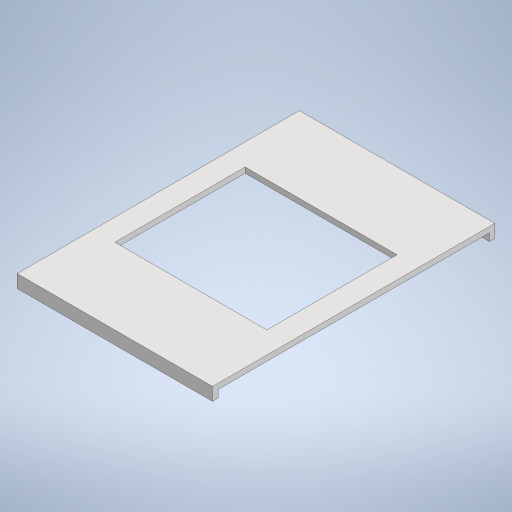
# Autodesk Inventor part: machine_platform
Saved by Autodesk Inventor 2024 (Build 280153000, 153)
## iProperties
Created: 2023-08-26
Part Number: machine_platform
Material: Generic
Document SubType Name: Modeling
Designer: l1534
Density: 1 g/cm^3
Appearance: Default
Author: l1534
Autodesk Inventor part; units mm, degrees
ref_plane "YZ Plane" through (0, 0, 0) normal (1, 0, 0) x (0, 1, 0)
ref_plane "XZ Plane" through (0, 0, 0) normal (0, 1, 0) x (-1, 0, 0)
ref_plane "XY Plane" through (0, 0, 0) normal (0, 0, 1) x (1, 0, 0)
sketch "Sketch1" plane through (0, 0, 0) normal (0, 1, 0) x (-1, 0, 0)
  line L0 (50.1781, 160.1313) -> (-129.8219, 160.1313)
  line L1 (-129.8219, 160.1313) -> (-129.8219, -99.8687)
  line L2 (-129.8219, -99.8687) -> (50.1781, -99.8687)
  line L3 (50.1781, -99.8687) -> (50.1781, 160.1313)
  point P0 (0, 0)
  dimension "d0" = 260
  dimension "d1" = 180
  constraints: 8 end point, 2 parallel, 1 horizontal, 1 perpendicular
  measures "d0" distance of L2.end L0.start
  measures "d1" distance of L1.end L2.end
extrude "Extrusion1" add sketch "Sketch1" along normal blind 5
sketch "Sketch2" plane through (0, 0, 0) normal (0, -1, 0) x (1, 0, 0)
  line L0 (129.8219, 160.1313) -> (129.8219, -99.8687) projected
  line L1 (-50.1781, -99.8687) -> (-50.1781, 160.1313) projected
  line L2 (129.8219, 160.1313) -> (-50.1781, 160.1313)
  line L3 (-50.1781, 160.1313) -> (-50.1781, 155.1313)
  line L4 (-50.1781, 155.1313) -> (129.8219, 155.1313)
  line L5 (129.8219, 155.1313) -> (129.8219, 160.1313)
  line L6 (129.8219, -99.8687) -> (-50.1781, -99.8687)
  line L7 (-50.1781, -99.8687) -> (-50.1781, -94.8687)
  line L8 (-50.1781, -94.8687) -> (129.8219, -94.8687)
  line L9 (129.8219, -94.8687) -> (129.8219, -99.8687)
  point P0 (0, 0)
  point P1 (129.8219, 155.1313)
  dimension "d4" = 5
  dimension "d5" = 5
  constraints: 16 end point, 4 parallel, 2 horizontal, 2 perpendicular, 2 point on line
  measures "d4" distance between parallel lines of L2 L4
  measures "d5" distance between parallel lines of L6 L8
extrude "Extrusion2" add sketch "Sketch2" along normal blind 7 contours L0 L4 L1 L2 | L0 L6 L1 L8
sketch "Sketch3" plane through (0, 5, 0) normal (0, 1, 0) x (1, 0, 0)
  line L0 (109.8219, 29.8687) -> (-30.1781, 29.8687)
  line L1 (-30.1781, 29.8687) -> (-30.1781, -90.1313)
  line L2 (-30.1781, -90.1313) -> (109.8219, -90.1313)
  line L3 (109.8219, -90.1313) -> (109.8219, 29.8687)
  line L4 (129.8219, -160.1313) -> (129.8219, 99.8687) projected
  line L5 (-50.1781, 99.8687) -> (-50.1781, -160.1313) projected
  line L6 (-50.1781, -160.1313) -> (129.8219, -160.1313) projected
  line L7 (129.8219, 99.8687) -> (-50.1781, 99.8687) projected
  point P0 (0, 0)
  dimension "d8" = 20
  dimension "d9" = 20
  dimension "d10" = 70
  dimension "d11" = 70
  constraints: 8 end point, 2 parallel, 1 horizontal, 1 perpendicular
  measures "d8" distance between parallel lines of L4 L3
  measures "d9" distance between parallel lines of L5 L1
  measures "d10" distance between parallel lines of L6 L2
  measures "d11" distance between parallel lines of L7 L0
extrude "Extrusion3" cut sketch "Sketch3" against normal through all contours L3 L2 L1 L0
body "Solid1"
